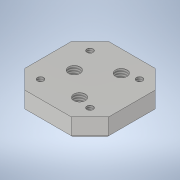
# Autodesk Inventor part: Platform A
Saved by Autodesk Inventor 2022 (Build 260153000, 153)
## iProperties
Created: 2021-01-07
Part Number: Platform A
Material: Generic
Document SubType Name: Modeling
Designer: caleb
Density: 1 g/cm^3
Appearance: Default
Author: caleb
Autodesk Inventor part; units mm, degrees
ref_plane "YZ Plane" through (0, 0, 0) normal (1, 0, 0) x (0, 1, 0)
ref_plane "XZ Plane" through (0, 0, 0) normal (0, 1, 0) x (-1, 0, 0)
ref_plane "XY Plane" through (0, 0, 0) normal (0, 0, 1) x (1, 0, 0)
sketch "Sketch1" plane through (0, 0, 0) normal (0, 1, 0) x (-1, 0, 0)
  line L0 (-14.2875, 14.2875) -> (14.2875, 14.2875)
  line L1 (14.2875, 14.2875) -> (14.2875, -14.2875)
  line L2 (14.2875, -14.2875) -> (-14.2875, -14.2875)
  line L3 (-14.2875, -14.2875) -> (-14.2875, 14.2875)
  line L4 (-14.2875, 14.2875) -> (14.2875, -14.2875) construction
  line L5 (14.2875, 14.2875) -> (-14.2875, -14.2875) construction
  point P0 (0, 0)
  dimension "d0" = 28.575
  dimension "d1" = 28.575
  constraints: 12 end point, 2 midpoint, 2 parallel, 1 horizontal, 1 perpendicular
  measures "d0" distance of L0.end L1.end
  measures "d1" distance of L0.start L0.end
extrude "Extrusion1" add sketch "Sketch1" along normal blind 6.35
sketch "Sketch6" plane through (0, 0, 0) normal (0, -1, 0) x (1, 0, 0)
  point P0 (0, 0)
  point P1 (3.556, 7.112)
  point P2 (3.556, -7.112)
  point P3 (-5.334, 0)
  dimension "d74" = 7.112
  dimension "d75" = 14.224
  dimension "d76" = 3.556
  dimension "d77" = 5.334
  constraints: 1 horizontal alignment, 1 vertical alignment
  measures "d74" vertical distance of point (3.556, 7.112) point (0, 0)
  measures "d75" distance of point (3.556, -7.112) point (3.556, 7.112)
  measures "d76" horizontal distance of point (3.556, 7.112) point (0, 0)
  measures "d77" distance of point (0, 0) point (-5.334, 0)
sketch "Sketch7" plane through (0, 6.35, 0) normal (0, 1, 0) x (1, 0, 0)
  circle A0 centre (-8.4201, -8.4201) radius 1.4986
  line L0 (-14.9987, 44.9961) -> (-14.9987, -44.9961)
  line L1 (-14.9987, -44.9961) -> (14.9987, -44.9961)
  circle A1 centre (-8.4201, 8.4201) radius 1.4986
  circle A2 centre (8.4201, -8.4201) radius 1.4986
  circle A3 centre (8.4201, 8.4201) radius 1.4986
  point P0 (0, 0)
  dimension "d62" = 2.9972
  dimension "d64" = 8.4201
  dimension "d57" = 16.8402
  dimension "d56" = 16.8402
  dimension "d63" = 8.4201
  constraints: 4 centre point, 4 end point, 1 horizontal, 1 vertical, 6 other
  measures "d62" diameter of A0
  measures "d64" horizontal distance of A0.centre point (0, 0)
  measures "d57" distance of A0.centre A1.centre
  measures "d56" distance of A0.centre A2.centre
  measures "d63" horizontal distance of point (0, 0) A0.centre
hole "Hole4" at (8.4201, 6.35, -8.4201) at (-8.4201, 6.35, -8.4201) at (-8.4201, 6.35, 8.4201) at (8.4201, 6.35, 8.4201) direction (0, -1, 0) diameter 2.159 depth 5.588 tip angle 118
hole "Hole5" at (3.556, 0, 7.112) at (3.556, 0, -7.112) at (-5.334, 0, 0) direction (0, 1, 0) diameter 3.9624 end through all thread size "10-32 UNF" class "2B" standard "ANSI Unified Screw Threads"
chamfer "Chamfer3" distance 6.35 angle 45 4 edges at (-14.2875, 3.175, 14.2875) (14.2875, 3.175, 14.2875) (14.2875, 3.175, -14.2875) (-14.2875, 3.175, -14.2875)
chamfer "Chamfer4" distance 0.7937 angle 45 8 edges at (0, 0, -14.2875) (11.1125, 0, -11.1125) (14.2875, 0, 0) (11.1125, 0, 11.1125) (0, 0, 14.2875) (-11.1125, 0, 11.1125) (-14.2875, 0, 0) (-11.1125, 0, -11.1125)
equation "\"d75\" = 2 * d74"
equation "\"d77\" = 1.5 * d76"
body "Solid1"
